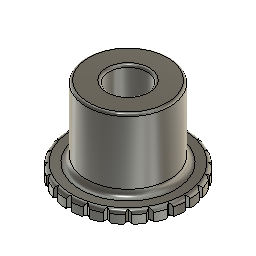
knob v7 (Autodesk Fusion 360 design; units mm, degrees)
Autodesk Fusion 360 part; units mm, degrees
sketch "Sketch1" plane through (0, 0, 0) normal (0, 0, 1) x (1, 0, 0)
  circle A0 centre (0, 0) radius 7
  circle A1 centre (0, 0) radius 3.2
  circle A2 centre (0, 0) radius 10
  dimension "d1" = 14
  dimension "d2" = 6.4
  dimension "d3" = 20
  constraint coincident A0.centre A1.centre
  constraint concentric A0 A1
  measures "d1" diameter of A0
  measures "d2" diameter of A1
  measures "d3" diameter of A2
extrude "Extrude1" add sketch "Sketch1" along normal blind 14 contours A0
extrude "Extrude2" add sketch "Sketch1" along normal blind 2 contours A2
extrude "Extrude3" add sketch "Sketch1" along normal blind 2 contours A1
ref_plane "WorkPlane1" through (0, 0, 12) normal (0, 0, -1) x (-1, 0, 0)
sketch "Sketch2" plane through (0, 0, 12) normal (0, 0, -1) x (-1, 0, 0)
  circle A0 centre (0, 0) radius 3.2
  circle A1 centre (0, 0) radius 7
  line L0 (-1.5, -4.2279) -> (-4.4448, -4.2279)
  line L1 (-4.4448, -4.2279) -> (-4.4448, 3.9067)
  line L2 (-4.4448, 3.9067) -> (-1.5, 3.9067)
  line L3 (-1.5, 3.9067) -> (-1.5, -4.2279)
  dimension "d10" = 1.5
  constraint horizontal L0
  constraint vertical L1
  constraint horizontal L2
  constraint vertical L3
  measures "d10" distance of A0.centre L3
extrude "Extrude4" add sketch "Sketch2" along normal blind 10 contours A0 L3 picked at (-2.0639, -0.0769)
fillet "Fillet1" radius 1 1 edges at (-6.5263, -2.5313, 2)
fillet "Fillet2" radius 0.4 3 edges at (-6.5263, -2.5313, 14) (1.5, 0, 12) (-2.9834, 1.1572, 14)
fillet "Fillet3" radius 0.6 1 edges at (-9.3233, -3.6162, 2)
sketch "Sketch3" plane through (0, 0, 0) normal (0, 0, -1) x (1, 0, 0)
  circle A0 centre (0, 0) radius 10
  line L0 (-0.3525, 9.9938) -> (0.0104, 9.5958)
  line L1 (0.0104, 9.5958) -> (0.443, 9.9902)
  constraint coincident A0 L0.start
  constraint coincident A0 L1.end
  constraint perpendicular L0 L1
extrude "Extrude5" cut sketch "Sketch3" against normal blind 2 contours A0 L0 L1 picked at (0.0337, 9.8646)
fillet "Fillet4" radius 0.2 2 edges at (-0.171, -9.7948, 0) (0.2267, -9.793, 0)
pattern_circular "C-Pattern1" count 24 over 360 about axis through (0, 0, 0) along (0, 0, 1) of "Extrude5", "Fillet4"
named bodies: "MIW knob"
